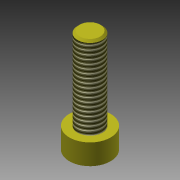
# Autodesk Inventor part: 砂轮轴端盖螺丝
Saved by Autodesk Inventor 2015 (Build 190159000, 159)
## iProperties
Created: 2017-05-16
Part Number: 砂轮轴端盖螺丝
Material: 常规
Document SubType Name: Modeling
Designer: Administrator
Density: 1 g/cm^3
Appearance: 淡黄色
Author: Administrator
Autodesk Inventor part; units mm, degrees
ref_plane "YZ Plane" through (0, 0, 0) normal (1, 0, 0) x (0, 1, 0)
ref_plane "XZ Plane" through (0, 0, 0) normal (0, 1, 0) x (-1, 0, 0)
ref_plane "XY Plane" through (0, 0, 0) normal (0, 0, 1) x (1, 0, 0)
sketch "草图1" plane through (0, 0, 0) normal (0, 0, 1) x (1, 0, 0)
  circle A0 centre (0, 0) radius 2.5
  dimension "d0" = 5
  constraints: 1 centre point, 1 coincident
  measures "d0" diameter of A0
extrude "拉伸1" add sketch "草图1" along normal blind 2.5
sketch "草图2" plane through (0, 0, 2.5) normal (0, 0, 1) x (1, 0, 0)
  circle A0 centre (0, 0) radius 1.5
  dimension "d3" = 3
  constraints: 1 centre point, 1 coincident
  measures "d3" diameter of A0
extrude "拉伸2" add sketch "草图2" along normal blind 10
thread "螺纹1" size "M3x0.5" class "6g" standard "ANSI Metric M Profile" full length
chamfer "倒角1" distance 0.25 angle 45 1 edges at (-1.5, 0, 12.5)
sketch "草图3" plane through (0, 0, 0) normal (0, 0, -1) x (-1, 0, 0)
  line L0 (0.866, -1.5) -> (-0.866, -1.5)
  line L1 (-0.866, -1.5) -> (-1.7321, 0)
  line L2 (-1.7321, 0) -> (-0.866, 1.5)
  line L3 (-0.866, 1.5) -> (0.866, 1.5)
  line L4 (0.866, 1.5) -> (1.7321, 0)
  line L5 (1.7321, 0) -> (0.866, -1.5)
  line L6 (0, 0) -> (0, 0.2895)
  circle A0 centre (0, 0) radius 1.5 projected
  point P0 (0, 1.5)
  dimension "d11" = 0.2895
  dimension "d12" = 1.5
  constraints: 14 end point, 1 coincident, 1 midpoint, 1 point on line, 1 vertical, 13 other
  measures "d11" distance of L6.start L6.end
  measures "d12" distance from line of A0.centre L0
extrude "拉伸3" cut sketch "草图3" against normal blind 1.25
